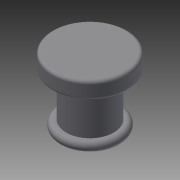
# Autodesk Inventor part: 2SS-R
Saved by Autodesk Inventor 2014 SP2 (Build 180246200, 246)
## iProperties
Created: 2018-12-09
Part Number: 2SS-R
Material: Generic
Catalog Web Link: www.cadenas.de
Description: 2 Series Stainless Steel Rivet-Capacitiy up to 325 lbs Each
Vendor: COLSONGROUP
Document SubType Name: Modeling
Designer: psadmin
Manufacturer: COLSONGROUP
Mass: 3.20107 g
Surface Area: 15.1225 cm^2
Volume: 3.20107 cm^3
Density: 1 g/cm^3
Appearance: PSOLRGB-175-175-175
Category: PARTsolutions
Company: COLSONGROUP
Title: 2SS-R
Author: Cadenas PARTsolutions
Comments: Capacitiy up to 325 lbs Each
PSOL_IDENT_0: {$CADENAS_DATA\23d-libs\colsongroup\colson\casters\2_series_stainless_steel\2_series_stainless_steel
PSOL_IDENT_1: _rivet.prj},174 {VTYP=3D},{NB=2SS-R},{LINA=2SS-R},{NN=2 Series Stainless Steel Rivet},{DATE=13.07.20
PSOL_IDENT_2: 17 07:15:59},{GEOMDATE=06.02.2017 10:23:00},{VERSION=},{LINEID=40},{WBVAR=},{WBNUMERIC=}  {NB=2SS-R}
PSOL_IDENT_3: ,{LINA=2SS-R},{KT=DUMMY},{PN=2SS-R}
NN: 2 Series Stainless Steel Rivet
NT: Capacitiy up to 325 lbs Each
NB: 2SS-R
NBSYN: $PN.
LINA: 2SS-R
PN: 2SS-R
SUPPLIER: COLSONGROUP
ARTICLENO: 2SS-R
BOMINFO: 2SS-R
CREATOR: CADENAS GmbH
Autodesk Inventor part; units mm, degrees
sketch "Sketch_1" plane through (0, 0, 0) normal (0, 0, 1) x (1, 0, 0)
  line L0 (0, -13.5382) -> (0, 4.4704)
  line L1 (0, 4.4704) -> (9.144, 4.4704)
  arc A0 (9.9314, 3.683) -> (9.144, 4.4704) centre (9.144, 3.683) ccw
  line L2 (9.9314, 3.683) -> (9.9314, 0.7874)
  arc A1 (9.144, 0) -> (9.9314, 0.7874) centre (9.144, 0.7874) ccw
  line L3 (9.144, 0) -> (6.6802, 0)
  arc A2 (6.6802, 0) -> (6.2738, -0.4064) centre (6.6802, -0.4064) ccw
  line L4 (6.2738, -0.4064) -> (6.2738, -11.1506)
  line L5 (6.2738, -11.1506) -> (6.8199, -11.1506)
  arc A3 (6.8199, -13.5382) -> (6.8199, -11.1506) centre (6.8199, -12.3444) ccw
  line L6 (6.8199, -13.5382) -> (0, -13.5382)
  line L7 (0, -13.5382) -> (0, 4.4704)
  constraints: 16 end point, 8 point on circle, 4 centre point
revolve "Revolution1" add sketch "Sketch_1" angle 360 about axis through (0, -13.5382, 0) along (0, -1, 0)
ref_plane "plate_rivet_XY" through (0, 0, 0) normal (0, -1, 0) x (1, 0, 0)
ref_plane "plate_rivet_YZ" through (0, 0, 0) normal (1, 0, 0) x (0, 0, 1)
ref_plane "plate_rivet_ZX" through (0, 0, 0) normal (0, 0, 1) x (0, -1, 0)
body "Solid1"
